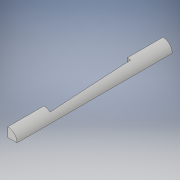
# Autodesk Inventor part: customMoulding
Saved by Autodesk Inventor 2019.1 (Build 231200000, 200)
## iProperties
Created: 2018-09-03
Part Number: customMoulding
Material: Generic
Document SubType Name: Modeling
Designer: steele
Density: 1 g/cm^3
Appearance: Default
Author: steele
Autodesk Inventor part; units mm, degrees
ref_plane "YZ Plane" through (0, 0, 0) normal (1, 0, 0) x (0, 1, 0)
ref_plane "XZ Plane" through (0, 0, 0) normal (0, 1, 0) x (-1, 0, 0)
ref_plane "XY Plane" through (0, 0, 0) normal (0, 0, 1) x (1, 0, 0)
sketch "Sketch1" plane through (0, 0, 0) normal (0, 0, 1) x (1, 0, 0)
  arc A0 (9.525, 0) -> (0, 9.525) centre (0, 0) ccw
  line L0 (0, 9.525) -> (0, 0)
  line L1 (0, 0) -> (9.525, 0)
  dimension "d0" = 19.05
  constraints: 4 end point, 2 point on circle, 1 centre point, 1 coincident, 1 perpendicular, 1 vertical
  measures "d0" diameter of A0
extrude "Extrusion1" add sketch "Sketch1" along normal mid plane 161.925
sketch "Sketch2" plane through (0, 0, 80.9625) normal (0, -1, 0) x (1, 0, 0)
  line L0 (0, -38.1) -> (6.35, -38.1)
  line L1 (3.175, -123.825) -> (0, -123.825)
  line L2 (0, -123.825) -> (0, -38.1)
  line L3 (9.525, -161.925) -> (0, -161.925) projected
  line L4 (0, -161.925) -> (0, 0) projected
  line L5 (3.175, -123.825) -> (6.35, -38.1)
  point P0 (0, -80.9625)
  dimension "d4" = 38.1
  dimension "d8" = 3.175
  dimension "d9" = 6.35
  constraints: 8 end point, 1 collinear, 1 horizontal, 1 parallel
  measures "d4" distance between parallel lines of L1 L3
  measures "d8" distance of L1.start L1.end
  measures "d9" distance of L0.start L0.end
extrude "Extrusion2" cut sketch "Sketch2" against normal through all
sketch "Sketch3" plane through (0, 0, -80.9625) normal (0, -1, 0) x (1, 0, 0)
  line L0 (9.525, 0) -> (0, 0) projected
  line L1 (0, 0) -> (0, 38.1) projected
  line L2 (9.525, 0) -> (0, 0)
  line L3 (0, 0) -> (0, 1.4732)
  line L4 (0, 1.4732) -> (9.525, 1.4732)
  line L5 (9.525, 1.4732) -> (9.525, 0)
  line L6 (0, 161.925) -> (9.525, 161.925) projected
  line L7 (9.525, 161.925) -> (9.525, 0) projected
  line L8 (0, 161.925) -> (9.525, 161.925)
  line L9 (9.525, 161.925) -> (9.525, 161.0106)
  line L10 (9.525, 161.0106) -> (0, 161.0106)
  line L11 (0, 161.0106) -> (0, 161.925)
  point P0 (0, 80.9625)
  dimension "d10" = 1.4732
  dimension "d11" = 0.9144
  constraints: 16 end point, 4 parallel, 2 horizontal, 2 perpendicular, 2 point on line
  measures "d10" distance between parallel lines of L0 L4
  measures "d11" distance between parallel lines of L10 L6
extrude "Extrusion3" cut sketch "Sketch3" against normal through all
equation "\"d0\" = cornerRoundType"
equation "\"d1\" = lengthOfPart"
equation "\"d4\" = bottomLength"
equation "\"d8\" = notchDepthLeftSide"
equation "\"d9\" = notchDepthRightSide"
equation "\"d10\" = leftSideLengthRemove"
equation "\"d11\" = rightSideLengthRemove"
equation "\"cornerRoundType\" = 19.05"
equation "\"notchCutout\" = 85.725"
equation "\"bottomLength\" = 38.1"
equation "\"lengthOfPart\" = 2 * bottomLength + notchCutout"
equation "\"notchDepth\" = 6.35"
equation "\"notchDepthLeftSide\" = 3.175"
equation "\"notchDepthRightSide\" = 6.35"
equation "\"leftSideLengthRemove\" = 1.4732"
equation "\"rightSideLengthRemove\" = 0.9144"
body "Solid1"
